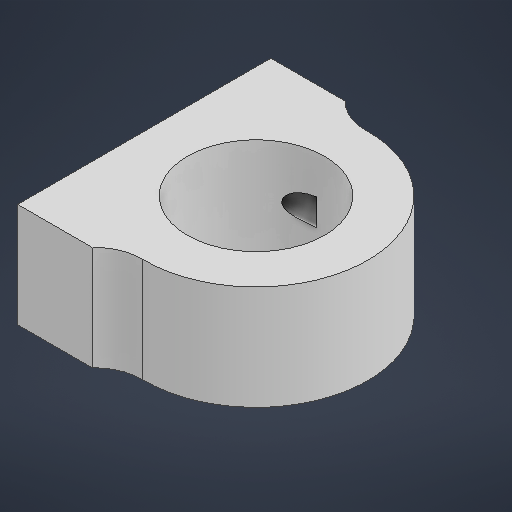
# Autodesk Inventor part: screw_support
Saved by Autodesk Inventor 2026.1 (Build 301233000, 233)
## iProperties
Created: 2025-09-23
Part Number: screw_support
Material: Generic
Document SubType Name: Modeling
Designer: emanuel
Density: 1 g/cm^3
Appearance: Default
Author: emanuel
Autodesk Inventor part; units mm, degrees
ref_plane "YZ Plane" through (0, 0, 0) normal (1, 0, 0) x (0, 1, 0)
ref_plane "XZ Plane" through (0, 0, 0) normal (0, 1, 0) x (-1, 0, 0)
ref_plane "XY Plane" through (0, 0, 0) normal (0, 0, 1) x (1, 0, 0)
sketch "Sketch1" plane through (0, 0, 0) normal (0, 1, 0) x (-1, 0, 0)
  circle A0 centre (0, 0) radius 4.6
  circle A1 centre (0, 0) radius 5.5
  line L0 (0, 5.5) -> (7.5, 5.5)
  line L1 (7.5, 5.5) -> (7.5, -5.5)
  line L2 (7.5, -5.5) -> (0, -5.5)
  line L3 (0, -5.5) -> (0, 5.5)
  line L4 (7.5, 5.5) -> (2.5, 5.5)
  line L5 (2.5, 5.5) -> (2.5, 8.5)
  line L6 (2.5, 8.5) -> (7.5, 8.5)
  line L7 (7.5, 8.5) -> (7.5, 5.5)
  line L8 (7.5, -5.5) -> (2.5, -5.5)
  line L9 (2.5, -5.5) -> (2.5, -8.5)
  line L10 (2.5, -8.5) -> (7.5, -8.5)
  line L11 (7.5, -8.5) -> (7.5, -5.5)
  circle A2 centre (0, 0) radius 7.5
  point P0 (2.5, -5.5)
  point P1 (2.5, 7.0711)
  point P2 (2.5, -7.0711)
  dimension "d1" = 11
  dimension "d0" = 9.2
  dimension "d2" = 5
  dimension "d3" = 3
  dimension "d4" = 5
  dimension "d5" = 3
  constraints: 24 end point, 6 parallel, 3 coincident, 3 horizontal, 3 perpendicular, 2 centre point, 3 other
  measures "d0" diameter of A0
  measures "d2" distance of L5.end L6.end
  measures "d3" distance of L4.end L5.end
  measures "d4" distance of L10.end L9.end
  measures "d5" distance of L9.end L8.end
extrude "Extrusion1" add sketch "Sketch1" along normal blind 7 contours A0 L3 A1 | A0 L3 A1 | L0 A2 L2 A1 | A1 L2 L9 A2 L5 L0 | L5 A2 L0 | L2 A2 L9 | A2 L5 L6 L7 L0 | L0 L1 A2 | A2 L1 L2 | L2 L11 L10 L9 A2
fillet "Fillet1" radius 3.175 2 edges at (-2.5, 3.5, -7.0711) (-2.5, 3.5, 7.0711)
sketch "Sketch2" plane through (-7.5, 0, -8.5) normal (-1, 0, 0) x (0, 0, 1)
  line L0 (0, 7) -> (17, 7) projected
  line L1 (0, 7) -> (3.5, 7)
  line L2 (3.5, 7) -> (13.5, 7)
  line L3 (3.5, 7) -> (3.5, 3.5)
  line L4 (0, 0) -> (17, 0) projected
  line L5 (13.5, 7) -> (13.5, 3.5)
  circle A0 centre (3.5, 3.5) radius 1
  circle A1 centre (13.5, 3.5) radius 1
  point P0 (8.5, 0)
  dimension "d9" = 3.5
  dimension "d10" = 10
  dimension "d11" = 3.5
  dimension "d12" = 3.5
  dimension "d13" = 2
  dimension "d14" = 2
  constraints: 8 end point, 2 centre point, 2 coincident, 2 point on line, 1 perpendicular, 1 vertical
  measures "d9" distance of L0.start L1.end
  measures "d10" distance of L1.end L2.end
  measures "d11" distance of L1.end L3.end
  measures "d12" distance of L2.end L5.end
  measures "d13" diameter of A0
  measures "d14" diameter of A1
extrude "Extrusion2" cut sketch "Sketch2" against normal blind 7
body "Solid1"
